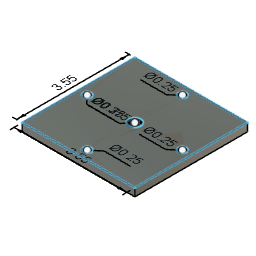
POWDER_Tx_Mount_Base_Plate_CAD_Model_v1 (Autodesk Fusion 360 design; units mm, degrees)
Autodesk Fusion 360 part; units mm, degrees
sketch "Sketch1" plane through (0, 0, 0) normal (0, 0, 1) x (1, 0, 0)
  circle A0 centre (0, -0.0368) radius 4.7625
  circle A1 centre (0, -38.1368) radius 3.175
  line L0 (-45.085, -45.1218) -> (45.085, -45.1218)
  line L1 (45.085, 45.0482) -> (-45.085, 45.0482)
  circle A2 centre (-38.1, -0.0368) radius 3.175
  line L2 (45.085, -45.1218) -> (45.085, 45.0482)
  circle A3 centre (38.1, -0.0368) radius 3.175
  line L3 (-45.085, 45.0482) -> (-45.085, -45.1218)
  circle A4 centre (0, 38.0632) radius 3.175
  circle A5 centre (0, -0.0368) radius 4.7625
  circle A6 centre (0, -38.1368) radius 3.175
  line L4 (-45.085, -45.1218) -> (45.085, -45.1218)
  line L5 (45.085, 45.0482) -> (-45.085, 45.0482)
  circle A7 centre (-38.1, -0.0368) radius 3.175
  line L6 (45.085, -45.1218) -> (45.085, 45.0482)
  circle A8 centre (38.1, -0.0368) radius 3.175
  line L7 (-45.085, 45.0482) -> (-45.085, -45.1218)
  circle A9 centre (0, 38.0632) radius 3.175
  dimension "d33" = 90.17
  dimension "d34" = 90.17
  dimension "d36" = 9.525
  dimension "d45" = 6.35
  dimension "d46" = 6.35
  dimension "d47" = 6.35
  dimension "d48" = 6.35
  dimension "d8" = 90.17
  dimension "d9" = 90.17
  dimension "d10" = 9.525
  dimension "d11" = 6.35
  dimension "d12" = 6.35
  dimension "d13" = 6.35
  dimension "d14" = 6.35
  constraint horizontal L0
  constraint vertical L2
  constraint horizontal L1
  constraint vertical L3
  constraint horizontal L4
  constraint vertical L6
  constraint horizontal L5
  constraint vertical L7
  measures "d33" distance of L1.end L0.start
  measures "d34" distance of L0.end L0.start
  measures "d36" diameter of A0
  measures "d45" diameter of A4
  measures "d46" diameter of A2
  measures "d47" diameter of A3
  measures "d48" diameter of A1
  measures "d8" distance of L1.end L0.start
  measures "d9" distance of L0.end L0.start
  measures "d10" diameter of A5
  measures "d11" diameter of A9
  measures "d12" diameter of A7
  measures "d13" diameter of A8
  measures "d14" diameter of A6
extrude "Extrude1" add sketch "Sketch1" against normal blind 6.35 in component "Base_Plate"
thread "Thread1" "ANSI Unified Screw Threads 0.25 1/4-20 UNC 3B" major diameter 6.35 minor diameter 5.1156 pitch 1.27 angle 60 modelled right hand crest width 0.3725 on face at (3.1592, 37.747, -4.2333) crest through (2.5578, 38.0632, -0.3175) in component "Base_Plate"
thread "Thread2" "ANSI Unified Screw Threads 0.25 1/4-20 UNC 3B" major diameter 6.35 minor diameter 5.1156 pitch 1.27 angle 60 modelled right hand crest width 0.3725 on face at (41.2592, -0.353, -4.2333) crest through (40.6578, -0.0368, -0.3175) in component "Base_Plate"
thread "Thread3" "ANSI Unified Screw Threads 0.25 1/4-20 UNC 3B" major diameter 6.35 minor diameter 5.1156 pitch 1.27 angle 60 modelled right hand crest width 0.3725 on face at (3.1592, -38.453, -4.2333) crest through (2.5578, -38.1368, -0.3175) in component "Base_Plate"
thread "Thread4" "ANSI Unified Screw Threads 0.25 1/4-20 UNC 3B" major diameter 6.35 minor diameter 5.1156 pitch 1.27 angle 60 modelled right hand crest width 0.3725 on face at (-34.9408, -0.353, -4.2333) crest through (-35.5422, -0.0368, -0.3175) in component "Base_Plate"
thread "Thread5" "ANSI Unified Screw Threads 0.375 3/8-16 UNC 3B" major diameter 9.525 minor diameter 7.94 pitch 1.5875 angle 60 modelled right hand crest width 0.4418 on face at (4.7388, -0.511, -4.2333) crest through (3.97, -0.0368, -0.3969) in component "Base_Plate"
component "Base_Plate" placed x (1, 0, 0) y (0, 1, 0) z (0, 0, 1) at (0, 0, 0)
